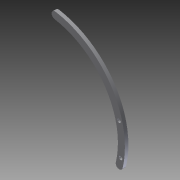
# Autodesk Inventor part: Disk Kicker v2
Saved by Autodesk Inventor 2012 (Build 160160000, 160)
## iProperties
Created: 2013-01-17
Part Number: Disk Kicker v2
Material: Default
Document SubType Name: Modeling
Designer: William
Density: 1 g/cm^3
Mass: 19.61 g
Surface Area: 97.0784 cm^2
Volume: 19.61 cm^3
Author: William
Autodesk Inventor part; units mm, degrees
ref_plane "YZ Plane" through (0, 0, 0) normal (1, 0, 0) x (0, 1, 0)
ref_plane "XZ Plane" through (0, 0, 0) normal (0, 1, 0) x (-1, 0, 0)
ref_plane "XY Plane" through (0, 0, 0) normal (0, 0, 1) x (1, 0, 0)
sketch "Sketch1" plane through (0, 0, 0) normal (0, 0, 1) x (1, 0, 0)
  arc A0 (135.8674, -32.4985) -> (24.2957, 137.5711) centre (0, 0) ccw
  arc A1 (148.2189, -35.4529) -> (26.5043, 150.0776) centre (0, 0) ccw
  arc A2 (135.8674, -32.4985) -> (148.2189, -35.4529) centre (142.0432, -33.9757) ccw
  arc A3 (26.5043, 150.0776) -> (24.2957, 137.5711) centre (25.4, 143.8243) ccw
  circle A4 centre (144.492, -21.2757) radius 3.175
  circle A5 centre (141.5755, 35.8743) radius 3.175
  dimension "d0" = 279.4
  dimension "d1" = 304.8
  dimension "d2" = 12.7
  dimension "d3" = 177.8
  dimension "d4" = 25.4
  dimension "d5" = 6.35
  dimension "d6" = 6.35
  dimension "d7" = 3.175
  dimension "d8" = 12.7
  dimension "d10" = 3.175
  dimension "d12" = 57.15
  constraints: 8 point on circle, 6 centre point, 3 tangent, 2 coincident
  measures "d0" diameter of A0
  measures "d1" diameter of A1
  measures "d2" diameter of A3
  measures "d3" vertical distance of A2.centre A3.centre
  measures "d4" horizontal distance of A3.centre point (0, 0)
  measures "d5" diameter of A4
  measures "d6" diameter of A5
  measures "d8" vertical distance of A2.centre A4.centre
  measures "d12" vertical distance of A4.centre A5.centre
extrude "Extrusion1" add sketch "Sketch1" along normal blind 6.35
body "Solid1"
